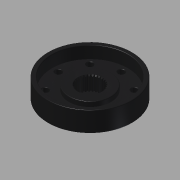
# Autodesk Inventor part: top-arm
Saved by Autodesk Inventor 2014 (Build 180170000, 170)
## iProperties
Created: 2013-07-13
Part Number: top-arm
Material: Generic
Document SubType Name: Modeling
Designer: Maurice
Density: 1 g/cm^3
Appearance: Default
Author: Maurice
Autodesk Inventor part; units mm, degrees
ref_plane "YZ Plane" through (0, 0, 0) normal (1, 0, 0) x (0, 1, 0)
ref_plane "XZ Plane" through (0, 0, 0) normal (0, 1, 0) x (-1, 0, 0)
ref_plane "XY Plane" through (0, 0, 0) normal (0, 0, 1) x (1, 0, 0)
sketch "Sketch1" plane through (0, 0, 0) normal (0, 1, 0) x (-1, 0, 0)
  circle A0 centre (0, 0) radius 10
  dimension "d0" = 20
  constraints: 1 centre point, 1 coincident
  measures "d0" diameter of A0
extrude "Extrusion1" add sketch "Sketch1" along normal blind 4.76
sketch "Sketch2" plane through (0, 0, 0) normal (0, -1, 0) x (1, 0, 0)
  circle A0 centre (0, 0) radius 10 projected
  circle A1 centre (0, 0) radius 5
  dimension "d3" = 10
  constraints: 1 centre point, 1 coincident
  measures "d3" diameter of A1
extrude "Extrusion2" add sketch "Sketch2" along normal blind 1 contours A1
sketch "Sketch3" plane through (0, 4.76, 0) normal (0, 1, 0) x (1, 0, 0)
  circle A0 centre (0, 0) radius 10 projected
  circle A1 centre (0, 0) radius 9
  dimension "d6" = 18
  constraints: 1 centre point, 1 coincident
  measures "d6" diameter of A1
extrude "Extrusion3" cut sketch "Sketch3" against normal blind 2.86 contours A1
sketch "Sketch4" plane through (0, 1.9, 0) normal (0, 1, 0) x (1, 0, 0)
  circle A0 centre (0, 0) radius 9 projected
  circle A1 centre (0, 0) radius 5
  dimension "d9" = 10
  constraints: 1 centre point, 1 coincident
  measures "d9" diameter of A1
extrude "Extrusion4" add sketch "Sketch4" along normal blind 1.13 contours A1
sketch "Sketch5" plane through (0, 3.03, 0) normal (0, 1, 0) x (1, 0, 0)
  circle A0 centre (0, 0) radius 5 projected
  circle A1 centre (0, 0) radius 2.935
  dimension "d12" = 5.87
  constraints: 1 centre point, 1 coincident
  measures "d12" diameter of A1
extrude "Extrusion5" cut sketch "Sketch5" against normal blind 3.37 contours A1
sketch "Sketch6" plane through (0, -0.34, 0) normal (0, 1, 0) x (1, 0, 0)
  circle A0 centre (0, 0) radius 2.935 projected
  circle A1 centre (0, 0) radius 2.68 construction
  line L0 (-0.1, -2.68) -> (0.1, -2.68)
  line L1 (-0.21, -2.935) -> (0, -2.935)
  line L2 (-0.21, -2.935) -> (-0.2069, -2.9277)
  line L3 (0.21, -2.935) -> (0.2069, -2.9277)
  arc A2 (-0.2069, -2.9277) -> (0.2069, -2.9277) centre (0, 0) ccw
  line L4 (-0.2069, -2.9277) -> (-0.1, -2.68)
  line L5 (0, -2.935) -> (0.21, -2.935)
  line L6 (0.2069, -2.9277) -> (0.1, -2.68)
  point P0 (0, -2.68)
  dimension "d15" = 5.36
  dimension "d16" = 0.2
  dimension "d17" = 0.42
  constraints: 14 end point, 6 point on circle, 3 vertical alignment, 2 parallel, 1 centre point, 1 coincident, 1 horizontal, 1 midpoint, 2 other
  measures "d16" distance of L0.start L0.end
  measures "d17" distance of L1.start L3.start
extrude "Extrusion6" add sketch "Sketch6" along normal up to surface (3.37 mm away) contours L4 L0 L6 A0 picked at (0, -2.765)
pattern_circular "Circular Pattern1" count 30 over 360 about axis through (0, -10, 0) along (0, 1, 0) of "Extrusion6"
sketch "Sketch7" plane through (0, 0, 0) normal (0, 0, 1) x (1, 0, 0)
  line L0 (-0.2069, 3.03) -> (-0.4064, 3.03) construction
  line L1 (-0.4594, 3.03) -> (-0.4064, 3.03) construction
  line L2 (-0.655, 3.03) -> (-0.4594, 3.03) construction
  line L3 (-0.811, 3.03) -> (-0.655, 3.03) construction
  line L4 (-0.811, 3.03) -> (-1.0018, 3.03) construction
  line L5 (-0.9987, 3.03) -> (-1.0018, 3.03) construction
  line L6 (-1.1814, 3.03) -> (-0.9987, 3.03) construction
  line L7 (-1.3798, 3.03) -> (-1.1814, 3.03) construction
  line L8 (-1.3798, 3.03) -> (-1.5535, 3.03) construction
  line L9 (-1.4944, 3.03) -> (-1.5535, 3.03) construction
  line L10 (-1.6562, 3.03) -> (-1.4944, 3.03) construction
  line L11 (-1.8882, 3.03) -> (-1.6562, 3.03) construction
  line L12 (-1.8882, 3.03) -> (-2.0373, 3.03) construction
  line L13 (-1.9247, 3.03) -> (-2.0373, 3.03) construction
  line L14 (-2.0585, 3.03) -> (-1.9247, 3.03) construction
  line L15 (-2.3141, 3.03) -> (-2.0585, 3.03) construction
  line L16 (-2.3141, 3.03) -> (-2.432, 3.03) construction
  line L17 (-2.2709, 3.03) -> (-2.432, 3.03) construction
  line L18 (-2.3709, 3.03) -> (-2.2709, 3.03) construction
  line L19 (-2.6389, 3.03) -> (-2.3709, 3.03) construction
  line L20 (-2.6389, 3.03) -> (-2.7205, 3.03) construction
  line L21 (-2.5179, 3.03) -> (-2.7205, 3.03) construction
  line L22 (-2.5797, 3.03) -> (-2.5179, 3.03) construction
  line L23 (-2.8483, 3.03) -> (-2.5797, 3.03) construction
  line L24 (-2.8483, 3.03) -> (-2.89, 3.03) construction
  line L25 (-2.6549, 3.03) -> (-2.89, 3.03) construction
  line L26 (-2.6758, 3.03) -> (-2.6549, 3.03) construction
  line L27 (-2.9333, 3.03) -> (-2.6758, 3.03) construction
  line L28 (-2.9333, 3.03) -> (-2.9333, 3.03) construction
  line L29 (-2.6758, 3.03) -> (-2.9333, 3.03) construction
  line L30 (-2.6549, 3.03) -> (-2.6758, 3.03) construction
  line L31 (-2.89, 3.03) -> (-2.6549, 3.03) construction
  line L32 (-2.89, 3.03) -> (-2.8483, 3.03) construction
  line L33 (-2.5797, 3.03) -> (-2.8483, 3.03) construction
  line L34 (-2.5179, 3.03) -> (-2.5797, 3.03) construction
  line L35 (-2.7205, 3.03) -> (-2.5179, 3.03) construction
  line L36 (-2.7205, 3.03) -> (-2.6389, 3.03) construction
  line L37 (-2.3709, 3.03) -> (-2.6389, 3.03) construction
  line L38 (-2.2709, 3.03) -> (-2.3709, 3.03) construction
  line L39 (-2.432, 3.03) -> (-2.2709, 3.03) construction
  line L40 (-2.432, 3.03) -> (-2.3141, 3.03) construction
  line L41 (-2.0585, 3.03) -> (-2.3141, 3.03) construction
  line L42 (-1.9247, 3.03) -> (-2.0585, 3.03) construction
  line L43 (-2.0373, 3.03) -> (-1.9247, 3.03) construction
  line L44 (-2.0373, 3.03) -> (-1.8882, 3.03) construction
  line L45 (-1.6562, 3.03) -> (-1.8882, 3.03) construction
  line L46 (-1.4944, 3.03) -> (-1.6562, 3.03) construction
  line L47 (-1.5535, 3.03) -> (-1.4944, 3.03) construction
  line L48 (-1.5535, 3.03) -> (-1.3798, 3.03) construction
  line L49 (-1.1814, 3.03) -> (-1.3798, 3.03) construction
  line L50 (-0.9987, 3.03) -> (-1.1814, 3.03) construction
  line L51 (-1.0018, 3.03) -> (-0.9987, 3.03) construction
  line L52 (-1.0018, 3.03) -> (-0.811, 3.03) construction
  line L53 (-0.655, 3.03) -> (-0.811, 3.03) construction
  line L54 (-0.4594, 3.03) -> (-0.655, 3.03) construction
  line L55 (-0.4064, 3.03) -> (-0.4594, 3.03) construction
  line L56 (-0.4064, 3.03) -> (-0.2069, 3.03) construction
  line L57 (-0.1, 3.03) -> (-0.2069, 3.03) construction
  line L58 (0.1, 3.03) -> (-0.1, 3.03) construction
  line L59 (0.2069, 3.03) -> (0.1, 3.03) construction
  line L60 (0.2069, 3.03) -> (0.4064, 3.03) construction
  line L61 (0.4594, 3.03) -> (0.4064, 3.03) construction
  line L62 (0.655, 3.03) -> (0.4594, 3.03) construction
  line L63 (0.811, 3.03) -> (0.655, 3.03) construction
  line L64 (0.811, 3.03) -> (1.0018, 3.03) construction
  line L65 (0.9987, 3.03) -> (1.0018, 3.03) construction
  line L66 (1.1814, 3.03) -> (0.9987, 3.03) construction
  line L67 (1.3798, 3.03) -> (1.1814, 3.03) construction
  line L68 (1.3798, 3.03) -> (1.5535, 3.03) construction
  line L69 (1.4944, 3.03) -> (1.5535, 3.03) construction
  line L70 (1.6562, 3.03) -> (1.4944, 3.03) construction
  line L71 (1.8882, 3.03) -> (1.6562, 3.03) construction
  line L72 (1.8882, 3.03) -> (2.0373, 3.03) construction
  line L73 (1.9247, 3.03) -> (2.0373, 3.03) construction
  line L74 (2.0585, 3.03) -> (1.9247, 3.03) construction
  line L75 (2.3141, 3.03) -> (2.0585, 3.03) construction
  line L76 (2.3141, 3.03) -> (2.432, 3.03) construction
  line L77 (2.2709, 3.03) -> (2.432, 3.03) construction
  line L78 (2.3709, 3.03) -> (2.2709, 3.03) construction
  line L79 (2.6389, 3.03) -> (2.3709, 3.03) construction
  line L80 (2.6389, 3.03) -> (2.7205, 3.03) construction
  line L81 (2.5179, 3.03) -> (2.7205, 3.03) construction
  line L82 (2.5797, 3.03) -> (2.5179, 3.03) construction
  line L83 (2.8483, 3.03) -> (2.5797, 3.03) construction
  line L84 (2.8483, 3.03) -> (2.89, 3.03) construction
  line L85 (2.6549, 3.03) -> (2.89, 3.03) construction
  line L86 (2.6758, 3.03) -> (2.6549, 3.03) construction
  line L87 (2.9333, 3.03) -> (2.6758, 3.03) construction
  line L88 (2.9333, 3.03) -> (2.9333, 3.03) construction
  line L89 (2.6758, 3.03) -> (2.9333, 3.03) construction
  line L90 (2.6549, 3.03) -> (2.6758, 3.03) construction
  line L91 (2.89, 3.03) -> (2.6549, 3.03) construction
  line L92 (2.89, 3.03) -> (2.8483, 3.03) construction
  line L93 (2.5797, 3.03) -> (2.8483, 3.03) construction
  line L94 (2.5179, 3.03) -> (2.5797, 3.03) construction
  line L95 (2.7205, 3.03) -> (2.5179, 3.03) construction
  line L96 (2.7205, 3.03) -> (2.6389, 3.03) construction
  line L97 (2.3709, 3.03) -> (2.6389, 3.03) construction
  line L98 (2.2709, 3.03) -> (2.3709, 3.03) construction
  line L99 (2.432, 3.03) -> (2.2709, 3.03) construction
  line L100 (2.432, 3.03) -> (2.3141, 3.03) construction
  line L101 (2.0585, 3.03) -> (2.3141, 3.03) construction
  line L102 (1.9247, 3.03) -> (2.0585, 3.03) construction
  line L103 (2.0373, 3.03) -> (1.9247, 3.03) construction
  line L104 (2.0373, 3.03) -> (1.8882, 3.03) construction
  line L105 (1.6562, 3.03) -> (1.8882, 3.03) construction
  line L106 (1.4944, 3.03) -> (1.6562, 3.03) construction
  line L107 (1.5535, 3.03) -> (1.4944, 3.03) construction
  line L108 (1.5535, 3.03) -> (1.3798, 3.03) construction
  line L109 (1.1814, 3.03) -> (1.3798, 3.03) construction
  line L110 (0.9987, 3.03) -> (1.1814, 3.03) construction
  line L111 (1.0018, 3.03) -> (0.9987, 3.03) construction
  line L112 (1.0018, 3.03) -> (0.811, 3.03) construction
  line L113 (0.655, 3.03) -> (0.811, 3.03) construction
  line L114 (0.4594, 3.03) -> (0.655, 3.03) construction
  line L115 (0.4064, 3.03) -> (0.4594, 3.03) construction
  line L116 (0.4064, 3.03) -> (0.2069, 3.03) construction
  line L117 (0.1, 3.03) -> (0.2069, 3.03) construction
  line L118 (-0.1, 3.03) -> (0.1, 3.03) construction
  line L119 (-0.2069, 3.03) -> (-0.1, 3.03) construction
  line L120 (5, 3.03) -> (-5, 3.03) construction
  line L121 (-2.935, 3.03) -> (-2.9333, 3.03) construction
  line L122 (-2.9333, -0.34) -> (-2.9333, 3.03) construction
  line L123 (-2.935, 3.03) -> (-3.6421, 3.7371)
  line L124 (-2.935, 3.03) -> (-1.935, 3.03) construction
  line L125 (-2.935, 3.03) -> (-2.2279, 2.3229)
  line L126 (-2.2279, 2.3229) -> (-2.2279, 3.03)
  line L127 (-2.2279, 3.03) -> (-2.935, 3.03)
  line L128 (0, -2.152) -> (0, 5.912) projected
  point P0 (0, 0)
  dimension "d23" = 1
  dimension "d24" = 135
  dimension "d25" = 1
  constraints: 10 end point, 2 collinear, 1 equal length, 1 horizontal, 1 perpendicular, 1 point on line
  measures "d23" distance of L121.start L123.end
  measures "d24" angle of L124 L123
  measures "d25" distance of L121.start L125.end
revolve "Revolution1" cut sketch "Sketch7" angle 360 about axis through (0, -10, 0) along (0, 1, 0)
sketch "Sketch8" plane through (0, -1, 0) normal (0, -1, 0) x (1, 0, 0)
  circle A0 centre (0, 0) radius 5 projected
  circle A1 centre (0, 0) radius 1.41
  circle A2 centre (0, -1.91) radius 0.4
  line L0 (-0.4, -1.91) -> (-0.4, -1.3521)
  line L1 (0.4, -1.91) -> (0.4, -1.3521)
  dimension "d27" = 2.82
  dimension "d28" = 0.8
  dimension "d29" = 1.91
  constraints: 4 end point, 4 point on circle, 2 centre point, 2 tangent, 1 coincident, 1 parallel, 1 vertical
  measures "d27" diameter of A1
  measures "d28" diameter of A2
  measures "d29" distance of A1.centre A2.centre
extrude "Extrusion7" cut sketch "Sketch8" against normal through all contours A1 | A1 L1 A2 L0 | A2
sketch "Sketch9" plane through (0, 0, 0) normal (0, -1, 0) x (1, 0, 0)
  circle A0 centre (0, 0) radius 5 projected
  point P0 (0, 7.5)
  point P1 (-5.3033, 5.3033)
  point P2 (-7.5, 0)
  point P3 (-5.3033, -5.3033)
  point P4 (0, -7.5)
  point P5 (5.3033, -5.3033)
  point P6 (7.5, 0)
  point P7 (5.3033, 5.3033)
  dimension "d32" = 7.5
  dimension "d35" = 360
  constraints: 1 vertical alignment, 9 other
  measures "d32" distance of A0.centre point (0, 7.5)
hole "Hole1" at (0, 0, 7.5) at (-5.3033, 0, 5.3033) at (-7.5, 0, 0) at (-5.3033, 0, -5.3033) at (0, 0, -7.5) at (5.3033, 0, -5.3033) at (7.5, 0, 0) at (5.3033, 0, 5.3033) direction (0, 1, 0) diameter 1.5 end through all
fillet "Fillet1" radius 0.15 5 edges at (10, 4.76, 0) (-9, 4.76, 0) (-5, 3.03, 0) (10, 0, 0) (-5, -1, 0)
chamfer "Chamfer1" distance 0.1 angle 45 16 edges at (-7.5, 1.9, 0.75) (-5.3033, 1.9, -4.5533) (0, 1.9, -6.75) (5.3033, 1.9, -4.5533) (7.5, 1.9, 0.75) (5.3033, 1.9, 6.0533) (0, 1.9, 8.25) (-5.3033, 1.9, 6.0533) (5.3033, 0, 6.0533) (0, 0, 8.25) (-5.3033, 0, 6.0533) (-7.5, 0, 0.75) (-5.3033, 0, -4.5533) (0, 0, -6.75) (5.3033, 0, -4.5533) (7.5, 0, 0.75)
body "Solid1"
